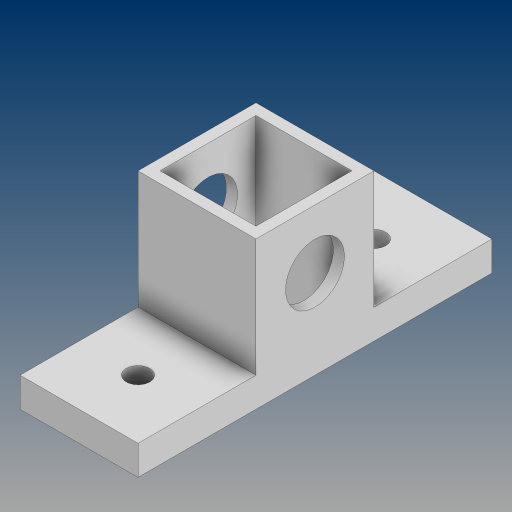
# Autodesk Inventor part: DragBarLinkage3 SingleBillet1
Saved by Autodesk Inventor 2024.3 (Build 283343000, 343)
## iProperties
Created: 2024-07-08
Part Number: DragBarLinkage3 SingleBillet1
Material: Generic
Document SubType Name: Modeling
Designer: Kenji
Density: 1 g/cm^3
Appearance: Default
Author: Kenji
Autodesk Inventor part; units mm, degrees
ref_plane "YZ Plane" through (0, 0, 0) normal (1, 0, 0) x (0, 1, 0)
ref_plane "XZ Plane" through (0, 0, 0) normal (0, 1, 0) x (-1, 0, 0)
ref_plane "XY Plane" through (0, 0, 0) normal (0, 0, 1) x (1, 0, 0)
sketch "Sketch1" plane through (0, 0, 0) normal (0, 1, 0) x (-1, 0, 0)
  line L0 (0, 0) -> (25.4, 0)
  line L1 (25.4, 0) -> (25.4, -76.2)
  line L2 (25.4, -76.2) -> (0, -76.2)
  line L3 (0, -76.2) -> (0, 0)
  circle A0 centre (12.7, -12.7) radius 2.54
  circle A1 centre (12.7, -63.5) radius 2.54
  line L4 (25.4, -25.4) -> (0, -25.4)
  line L5 (0, -25.4) -> (0, -50.8)
  line L6 (0, -50.8) -> (25.4, -50.8)
  line L7 (25.4, -50.8) -> (25.4, -25.4)
  point P0 (12.7, 0)
  point P1 (12.7, -76.2)
  dimension "d2" = 25.4
  dimension "d3" = 76.2
  dimension "d4" = 5.08
  dimension "d5" = 5.08
  dimension "d6" = 25.4
  dimension "d7" = 25.4
  dimension "d8" = 12.7
  dimension "d9" = 12.7
  constraints: 16 end point, 4 parallel, 2 centre point, 2 horizontal, 2 midpoint, 2 perpendicular, 2 point on line, 2 vertical alignment
  measures "d2" distance of L1.end L2.end
  measures "d3" distance of L0.end L1.end
  measures "d4" diameter of A0
  measures "d5" diameter of A1
  measures "d6" distance of L5.end L4.end
  measures "d7" distance of L4.start L0.end
  measures "d8" distance of point (12.7, -76.2) A1.centre
  measures "d9" distance of point (12.7, 0) A0.centre
extrude "Extrusion1" add sketch "Sketch1" along normal blind 6.35
sketch "Sketch2" plane through (0, 6.35, 0) normal (0, 1, 0) x (1, 0, 0)
  line L0 (0, 0) -> (0, 76.2) projected
  line L1 (0, 76.2) -> (-25.4, 76.2) projected
  line L2 (-25.4, 76.2) -> (-25.4, 0) projected
  line L3 (-25.4, 0) -> (0, 0) projected
  circle A0 centre (-12.7, 63.5) radius 2.54 projected
  circle A1 centre (-12.7, 12.7) radius 2.54 projected
  line L4 (-25.4, 76.2) -> (-25.4, 0) construction
  line L5 (0, 0) -> (0, 76.2) construction
  line L6 (-25.4, 0) -> (0, 0) construction
  line L7 (0, 0) -> (0, 76.2) construction
  line L8 (0, 76.2) -> (-25.4, 76.2) construction
  line L9 (-25.4, 76.2) -> (-25.4, 0) construction
  line L10 (-25.4, 25.4) -> (0, 25.4)
  line L11 (0, 25.4) -> (0, 50.8)
  line L12 (0, 50.8) -> (-25.4, 50.8)
  line L13 (-25.4, 50.8) -> (-25.4, 25.4)
  dimension "d12" = 25.4
  dimension "d13" = 25.4
  dimension "d14" = 25.4
  constraints: 16 end point, 4 parallel, 2 horizontal, 2 perpendicular, 1 point on line
  measures "d12" distance of L12.end L11.end
  measures "d13" distance of L11.end L10.end
  measures "d14" distance of L2.end L10.start
extrude "Extrusion2" add sketch "Sketch2" along normal blind 25.4 contours L10 L2 L12 L0
sketch "Sketch3" plane through (0, 0, 0) normal (1, 0, 0) x (0, 0, -1)
  line L0 (0, 0) -> (76.2, 0) projected
  line L1 (76.2, 0) -> (76.2, 6.35) projected
  line L2 (50.8, 6.35) -> (76.2, 6.35) projected
  line L3 (50.8, 6.35) -> (50.8, 31.75) projected
  line L4 (25.4, 31.75) -> (50.8, 31.75) projected
  line L5 (25.4, 6.35) -> (25.4, 31.75) projected
  line L6 (0, 6.35) -> (25.4, 6.35) projected
  line L7 (0, 0) -> (0, 6.35) projected
  point P0 (38.1, 19.05)
  point P1 (25.4, 19.05)
  point P2 (38.1, 31.75)
  dimension "d17" = 12.7
  dimension "d18" = 12.7
  constraints: 2 midpoint
  measures "d17" distance of point (25.4, 19.05) point (38.1, 19.05)
  measures "d18" distance of point (38.1, 31.75) point (38.1, 19.05)
hole "Hole1" at (0, 19.05, -38.1) direction (-1, 0, 0) diameter 12.7 end through all
sketch "Sketch4" plane through (0, 31.75, 0) normal (0, 1, 0) x (1, 0, 0)
  line L0 (-25.4, 50.8) -> (-25.4, 25.4) projected
  line L1 (-25.4, 25.4) -> (0, 25.4) projected
  line L2 (0, 25.4) -> (0, 50.8) projected
  line L3 (0, 50.8) -> (-25.4, 50.8) projected
  line L4 (-23.0188, 48.4188) -> (-23.0187, 27.7812)
  line L5 (-23.0187, 27.7812) -> (-2.3813, 27.7812)
  line L6 (-2.3813, 27.7812) -> (-2.3813, 48.4188)
  line L7 (-2.3813, 48.4188) -> (-23.0188, 48.4188)
  point P0 (0, 0)
  dimension "d26" = 2.3813
  constraints: 8 end point, 3 other
  measures "d26" distance between parallel lines of L3 L7
extrude "Extrusion3" cut sketch "Sketch4" against normal blind 31.75 contours L7 L6 L5 L4
body "Solid1"
